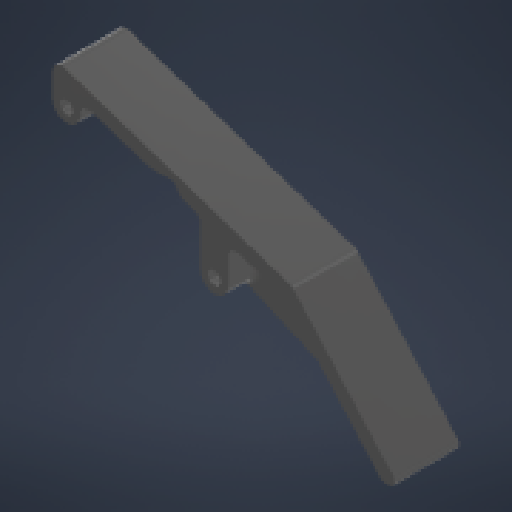
# Autodesk Inventor part: funnel
Saved by Autodesk Inventor 2025.2 (Build 292293000, 293)
## iProperties
Created: 2025-11-17
Part Number: funnel
Material: white pla
Document SubType Name: Modeling
Designer: cloudy
Density: 1 g/cm^3
Appearance: Smooth - Dark Gray
Author: cloudy
Autodesk Inventor part; units mm, degrees
ref_plane "YZ Plane" through (0, 0, 0) normal (1, 0, 0) x (0, 1, 0)
ref_plane "XZ Plane" through (0, 0, 0) normal (0, 1, 0) x (-1, 0, 0)
ref_plane "XY Plane" through (0, 0, 0) normal (0, 0, 1) x (1, 0, 0)
sketch "Sketch1" plane through (0, 0, 0) normal (0, 0, 1) x (1, 0, 0)
  circle A0 centre (-50.0249, 184.15) radius 2.1844 projected
  circle A1 centre (0.7751, 158.75) radius 2.1844 projected
  line L0 (-38.2655, 111.5928) -> (-11.4178, 111.5928) construction
  line L1 (-11.4178, 111.5928) -> (-11.4178, 180.5072)
  line L2 (-11.4178, 180.5072) -> (-38.2655, 180.5072)
  line L3 (-38.2655, 180.5072) -> (-38.2655, 111.5928) construction
  line L4 (-38.2655, 111.5928) -> (-11.4178, 180.5072) construction
  line L5 (-11.4178, 111.5928) -> (-38.2655, 180.5072) construction
  line L6 (-59.6662, -167.8681) -> (-59.6662, 213.1319) construction
  circle A2 centre (-50.0249, 184.15) radius 4.7625
  line L7 (-45.2624, 188.3316) -> (-3.9874, 174.6153)
  circle A3 centre (0.7751, 158.75) radius 4.7625
  line L8 (-3.9874, 158.75) -> (-3.9874, 174.6153)
  line L9 (27.4814, 169.5109) -> (-54.7874, 196.85)
  line L10 (-45.2624, 184.15) -> (-45.2624, 188.3316)
  line L11 (-54.7874, 184.15) -> (-54.7874, 196.85)
  line L12 (-54.7874, 196.85) -> (15.9837, 173.3318)
  line L13 (5.5376, 158.75) -> (5.5376, 171.45)
  line L14 (27.4814, 169.5109) -> (65.2478, 127)
  line L15 (65.2478, 127) -> (58.4526, 127)
  line L16 (58.4526, 127) -> (24.5876, 165.1194)
  line L17 (5.5376, 171.45) -> (24.5876, 165.1194)
  line L18 (107.7853, 127) -> (46.3173, 127) projected
  point P0 (0, 0)
  point P1 (-24.8417, 146.05)
  point P2 (-21.7175, 180.5072)
  point P3 (-11.4178, 177.0845)
  dimension "d1" = 381
  dimension "d2" = 9.525
  dimension "d4" = 9.525
  dimension "d5" = 5.08
  dimension "d6" = 12.7
  dimension "d7" = 12.7
  dimension "d8" = 150
  dimension "d9" = 5.08
  dimension "d10" = 19.05
  constraints: 36 end point, 6 vertical, 4 parallel, 4 point on circle, 4 tangent, 3 collinear, 3 horizontal, 2 centre point, 2 coincident, 2 midpoint, 1 perpendicular, 1 other
  measures "d1" distance of L6.start L6.end
  measures "d2" diameter of A2
  measures "d4" diameter of A3
  measures "d5" distance between parallel lines of L12 L7
  measures "d6" distance of L13.start L13.end
  measures "d7" distance of L9.end L11.start
  measures "d8" angle of L16 L17
  measures "d9" distance between parallel lines of L14 L16
  measures "d10" distance from line of L13 L16.end
extrude "Extrusion1" add sketch "Sketch1" along normal blind 22.225 contours L1 L2 L7 L10 A2 L11 L9 L14 L15 L16 L17 L13 A3 L8 | A3 | A2
fillet "Fillet1" radius 3.175 7 edges at (-54.7874, 196.85, 11.1125) (-45.2624, 188.3316, 11.1125) (-3.9874, 174.6153, 11.1125) (5.5376, 171.45, 11.1125) (24.5876, 165.1194, 11.1125) (27.4814, 169.5109, 11.1125) (58.4526, 127, 11.1125)
fillet "Fillet2" radius 2 1 edges at (65.2478, 127, 11.1125)
ref_plane "Work Plane1" through (0, 0, 11.1125) normal (0, 0, 1) x (1, 0, 0)
sketch "Sketch2" plane through (0, 0, 11.1125) normal (0, 0, 1) x (1, 0, 0)
  line L0 (5.5376, 158.75) -> (5.5376, 167.0492) construction
  line L1 (-1.1751, 154.4051) -> (57.5053, 128.0663)
  line L2 (25.1527, 164.4834) -> (57.5053, 128.0663) construction
  arc A0 (-3.9874, 158.75) -> (5.5376, 158.75) centre (0.7751, 158.75) ccw projected
  point P0 (0, 0)
  constraints: 2 end point, 1 point on circle, 1 tangent
extrude "Rib1" add sketch "Sketch2" along normal mid plane 2.54 rib yes fills toward (28.1856, 141.2813) open curves L1
fillet "Fillet3" radius 2 10 edges at (6.855, 169.624, 12.3825) (16.7471, 167.7249, 12.3825) (24.526, 165.0259, 12.3825) (41.329, 146.2749, 12.3825) (5.5376, 162.8996, 12.3825) (6.855, 169.624, 9.8425) (16.7471, 167.7249, 9.8425) (24.526, 165.0259, 9.8425) (41.329, 146.2749, 9.8425) (5.5376, 162.8996, 9.8425)
fillet "Fillet4" radius 12.7 1 edges at (-21.7175, 180.5072, 11.1125)
fillet "Fillet5" radius 3 2 edges at (-11.4178, 180.5072, 11.1125) (-11.4178, 177.0845, 11.1125)
body "Solid1"
